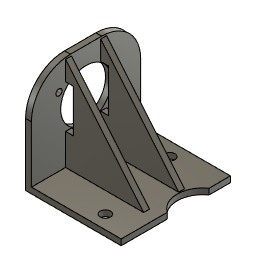
Roller+em+ferro (Autodesk Fusion 360 design; units mm, degrees)
Autodesk Fusion 360 part; units mm, degrees
note: some values were not read from the file. Set by a fixed rule: which sketch regions a step uses.
sketch "Esboço1" plane through (0, 0, 0) normal (0, 1, 0) x (1, 0, 0)
  line L0 (0, 0) -> (49, 0)
  line L1 (49, -56) -> (0, -56)
  line L2 (0, -56) -> (0, 0)
  line L3 (0, -28) -> (45.0349, -28)
  arc A0 (49, -11.0003) -> (49, -32.3769) centre (56.4, -21.6886) ccw
  line L4 (49, 0) -> (49, -11.0003)
  line L5 (49, -32.3769) -> (49, -56)
  circle A1 centre (24.93, -7) radius 2.65
  circle A2 centre (33.9, -49) radius 2.65
  dimension "d1" = 49
  dimension "d2" = 56
  dimension "d3" = 26
  dimension "d5" = 5.3
  dimension "d6" = 24.93
  dimension "d7" = 21
  dimension "d8" = 5.3
  dimension "d9" = 21
  dimension "d10" = 33.9
  dimension "d47" = 56.4
  constraint horizontal L0
  constraint vertical L4
  constraint horizontal L1
  constraint vertical L2
  constraint coincident L0.start L2.end
  constraint midpoint L2 L3.start
  constraint coincident A0.end L4
  constraint collinear L4 L5
  constraint coincident A0 L3.end
  measures "d1" distance of L0.start L0.end
  measures "d2" distance of L0.start L1.end
  measures "d3" diameter of A0
  measures "d5" diameter of A1
  measures "d6" distance of L2 A1.centre
  measures "d7" distance of L3 A1.centre
  measures "d8" diameter of A2
  measures "d9" distance of L3 A2.centre
  measures "d10" distance of L2 A2.centre
  measures "d47" distance of L2 A0.centre
extrude "Extrusão1" add sketch "Esboço1" along normal blind 3
sketch "Esboço2" plane through (0, 3, 0) normal (0, 1, 0) x (-1, 0, 0)
  circle A0 centre (-24.93, 7) radius 2.65
  circle A1 centre (-33.9, 49) radius 2.65
  arc A2 (-49, 11.0003) -> (-49, 32.3769) centre (-56.4, 21.6886) ccw
  line L0 (-49, 11.0003) -> (-49, 0)
  line L1 (-49, 0) -> (0, 0)
  line L2 (0, 0) -> (0, 56)
  line L3 (0, 56) -> (-49, 56)
  line L4 (-49, 56) -> (-49, 32.3769)
  line L5 (0, 0) -> (-3, 0)
  line L6 (-3, 0) -> (-3, 56)
  line L7 (-3, 56) -> (0, 56)
  line L8 (0, 56) -> (0, 0)
  constraint horizontal L5
  constraint vertical L6
  constraint horizontal L7
  constraint vertical L8
  constraint coincident L3 L6.end
  constraint coincident L1.end L2.start
extrude "Extrusão2" add sketch "Esboço2" along normal blind 49 contours L1 L2 L3 L5 L6 L7 L8
sketch "Esboço3" plane through (0, 0, 0) normal (-1, 0, 0) x (0, 0, 1)
  line L0 (0, 0) -> (56, 0)
  line L1 (56, 0) -> (56, 52)
  line L2 (56, 52) -> (0, 52)
  line L3 (0, 52) -> (0, 0)
  circle A0 centre (28, 30) radius 13
  circle A1 centre (28, 14) radius 1.6
  circle A2 centre (14.1436, 38) radius 1.6
  circle A3 centre (41.8564, 38) radius 1.6
  dimension "d15" = 26
  dimension "d16" = 30
  dimension "d19" = 3.2
  dimension "d20" = 16
  dimension "d21" = 8
  dimension "d22" = 13.8564
  measures "d15" diameter of A0
  measures "d16" distance of L0 A0.centre
  measures "d19" diameter of A1
  measures "d20" distance of A0.centre A1.centre
  measures "d21" vertical distance of A0.centre A3.centre
  measures "d22" horizontal distance of A0.centre A3.centre
ref_plane "Plano de trabalho1" through (0, 0, 19) normal (0, 0, 1) x (1, 0, 0)
sketch "Esboço4" plane through (0, 0, 19) normal (0, 0, 1) x (1, 0, 0)
  line L0 (3, 3) -> (43, 3)
  line L1 (43, 3) -> (3, 51)
  line L2 (3, 41) -> (7, 41)
  line L3 (7, 41) -> (7, 19)
  line L4 (7, 19) -> (3, 19)
  line L5 (3, 51) -> (3, 41)
  line L6 (3, 19) -> (3, 3)
  dimension "d26" = 40
  dimension "d27" = 48
  dimension "d39" = 10
  dimension "d40" = 32
  dimension "d41" = 4
  constraint horizontal L0
  constraint perpendicular L0 L5
  constraint perpendicular L2 L5
  constraint perpendicular L2 L3
  constraint coincident L4.end L5
  constraint perpendicular L4 L5
  constraint collinear L5 L6
  measures "d26" distance of L0.start L0.end
  measures "d27" distance of L0.start L1.end
  measures "d39" distance of L1.end L2
  measures "d40" distance of L1.end L4
  measures "d41" distance of L2.start L2.end
extrude "Extrusão4" add sketch "Esboço4" along normal blind 1.5 and the other way blind 1.5
ref_plane "Plano de trabalho2" through (0, 0, 37) normal (0, 0, 1) x (1, 0, 0)
sketch "Esboço5" plane through (0, 0, 37) normal (0, 0, 1) x (1, 0, 0)
  line L0 (3, 3) -> (43, 3)
  line L1 (43, 3) -> (3, 51)
  line L2 (3, 41) -> (7, 41)
  line L3 (7, 41) -> (7, 19)
  line L4 (7, 19) -> (3, 19)
  line L5 (3, 51) -> (3, 41)
  line L6 (3, 19) -> (3, 3)
  dimension "d29" = 40
  dimension "d30" = 48
  dimension "d42" = 10
  dimension "d43" = 32
  dimension "d44" = 4
  constraint vertical L5
  constraint perpendicular L0 L5
  constraint perpendicular L2 L5
  constraint perpendicular L2 L3
  constraint coincident L4.end L5
  constraint perpendicular L4 L5
  constraint collinear L5 L6
  measures "d29" distance of L0.start L0.end
  measures "d30" distance of L1.end L0.start
  measures "d42" distance of L1.end L2
  measures "d43" distance of L1.end L4
  measures "d44" distance of L2.start L2.end
extrude "Extrusão5" add sketch "Esboço5" along normal blind 1.5 and the other way blind 1.5
extrude "Extrusão3" cut sketch "Esboço3" against normal blind 6.5 contours A0 | A1 | A2 | A3
fillet "Arredondamento1" radius 20 2 edges at (1.5, 52, 56) (1.5, 52, 0)
